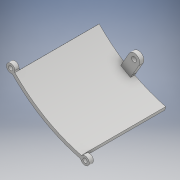
# Autodesk Inventor part: Wheel Guard1
Saved by Autodesk Inventor 2018 (Build 220112000, 112)
## iProperties
Created: 2017-10-13
Part Number: Wheel Guard1
Material: Generic
Document SubType Name: Modeling
Designer: BrisbaneMatt
Density: 1 g/cm^3
Appearance: Default
Author: BrisbaneMatt
Autodesk Inventor part; units mm, degrees
ref_plane "YZ Plane" through (0, 0, 0) normal (1, 0, 0) x (0, 1, 0)
ref_plane "XZ Plane" through (0, 0, 0) normal (0, 1, 0) x (-1, 0, 0)
ref_plane "XY Plane" through (0, 0, 0) normal (0, 0, 1) x (1, 0, 0)
sketch "Sketch1" plane through (0, 0, 0) normal (0, 1, 0) x (-1, 0, 0)
  circle A0 centre (0, 0) radius 100.151
  line L0 (0, 0) -> (50.0755, -86.7333)
  line L1 (0, 0) -> (100.151, 0) construction
  line L2 (0, 0) -> (50.0755, 86.7333)
  line L3 (0, 0) -> (100.151, 0) construction
  line L4 (0, 0) -> (-100.151, 0)
  line L5 (50.0755, -86.7333) -> (100.0755, -86.7333) construction
  line L6 (50.0755, -86.7333) -> (24.5339, -97.0995)
  line L7 (50.0755, -86.7333) -> (100.0755, -86.7333) construction
  line L8 (71.8237, -69.7967) -> (50.0755, -86.7333)
  circle A1 centre (0, 0) radius 102.651
  line L9 (0, 0) -> (71.8237, -69.7967)
  line L10 (71.8237, -69.7967) -> (73.6166, -71.539)
  line L11 (0, 0) -> (24.5339, -97.0995)
  line L12 (24.5339, -97.0995) -> (25.1463, -99.5233)
  dimension "d0" = 200.302
  dimension "d1" = 60
  dimension "d2" = 60
  dimension "d8" = 205.302
  constraints: 26 end point, 7 point on circle, 5 horizontal, 2 centre point, 2 coincident, 2 equal length, 2 point on line
  measures "d0" diameter of A0
  measures "d1" angle of L0 L1
  measures "d2" angle of L3 L2
  measures "d8" diameter of A1
extrude "Extrusion1" add sketch "Sketch1" along normal blind 40 contours L10 A1 L12 A0 picked at (67.2642, -76.2102)
sketch "Sketch2" plane through (0, 0, 0) normal (0, -1, 0) x (1, 0, 0)
  line L0 (-24.5339, -97.0995) -> (-25.1463, -99.5233) projected
  line L1 (-24.8401, -98.3114) -> (-21.9315, -99.0463)
  circle A0 centre (-21.9315, -99.0463) radius 1.5
  line L2 (-73.6166, -71.539) -> (-71.8237, -69.7967) projected
  line L3 (-72.7201, -70.6679) -> (-74.8716, -72.7586)
  line L4 (-74.8716, -72.7586) -> (-72.7201, -70.6679)
  line L5 (-72.7201, -70.6679) -> (-74.8109, -68.5164)
  circle A1 centre (-74.8109, -68.5164) radius 1.5
  circle A2 centre (-74.8109, -68.5164) radius 3
  arc A3 (-73.6166, -71.539) -> (-25.1463, -99.5233) centre (0, 0) ccw projected
  line L6 (-73.6166, -71.539) -> (-74.8109, -71.5164)
  arc A4 (-71.8237, -69.7967) -> (-24.5339, -97.0995) centre (0, 0) ccw projected
  line L7 (-71.8109, -68.5164) -> (-71.8237, -69.7967)
  circle A5 centre (-21.9315, -99.0463) radius 3
  line L8 (-21.9315, -99.0463) -> (-24.5296, -100.5463)
  line L9 (-21.9315, -99.0463) -> (-18.9315, -99.0463) construction
  line L10 (-24.5296, -100.5463) -> (-25.1463, -99.5233)
  arc A6 (-22.1585, -98.9889) -> (-21.9315, -99.0463) centre (-21.9315, -98.5684) ccw
  line L11 (-21.9315, -99.0463) -> (-22.9003, -97.4384)
  line L12 (-21.9315, -99.0463) -> (-20.0543, -99.0463) construction
  line L13 (-22.9003, -97.4384) -> (-23.4798, -96.4767)
  line L14 (-23.4798, -96.4767) -> (-24.5339, -97.0995)
  point P0 (0, 0)
  dimension "d12" = 3
  dimension "d13" = 3
  dimension "d14" = 3
  dimension "d15" = 210
  dimension "d16" = 121.07
  constraints: 26 end point, 8 point on circle, 5 centre point, 4 coincident, 2 collinear, 2 equal length, 2 horizontal, 2 midpoint, 2 point on line, 1 perpendicular, 1 tangent
  measures "d12" distance of L1.start L1.end
  measures "d13" distance of L3.start L3.end
  measures "d14" distance of L3.start L5.end
  measures "d16" angle of L12 L11
extrude "Extrusion2" add sketch "Sketch2" against normal blind 3 contours L14 A5 L0 | L7 L2 A2 | A5 L10 L0 | A5 L13 L11 A0 L1 | L1 A0 L8 A5 | A5 L8 A0 L11 L13 | A0 L11 L1 | L1 A6 L8 A0 | L2 L6 A2 | A2 | L1 A6 | A0 L8 L11
sketch "Sketch3" plane through (0, 3, 0) normal (0, 1, 0) x (1, 0, 0)
  arc A0 (-23.4798, 96.4767) -> (-24.5296, 100.5463) centre (-21.9315, 99.0463) ccw projected
  circle A1 centre (-21.9315, 99.0463) radius 1.5
  point P0 (0, 0)
  dimension "d19" = 3
  constraints: 1 centre point, 1 coincident
  measures "d19" diameter of A1
extrude "Extrusion3" cut sketch "Sketch3" against normal blind 3
sketch "Sketch4" plane through (-25.1463, 3, -99.5233) normal (0.9695, 0, -0.245) x (-0.245, 0, -0.9695)
  point P0 (-102.651, -3)
sketch "Sketch5" plane through (0, 40, 0) normal (0, 1, 0) x (1, 0, 0)
  circle A0 centre (-74.8109, 68.5164) radius 1.5 projected
  circle A1 centre (-21.9315, 99.0463) radius 1.5 projected
  line L0 (-74.8109, 68.5164) -> (-21.9315, 99.0463)
  circle A2 centre (-48.3712, 83.7814) radius 1.75
  circle A3 centre (-48.3712, 83.7814) radius 4
  line L1 (-44.9071, 85.7814) -> (-46.5714, 88.6641)
  arc A4 (-24.5339, 97.0995) -> (-71.8237, 69.7967) centre (0, 0) ccw projected
  line L2 (-51.8353, 81.7814) -> (-53.4996, 84.6641)
  line L3 (-46.5714, 88.6641) -> (-50.0755, 88.3957)
  line L4 (-50.0755, 88.3957) -> (-52.8557, 86.4967)
  line L5 (-52.8557, 86.4967) -> (-53.4996, 84.6641)
  point P0 (0, 0)
  dimension "d22" = 3.5
  dimension "d23" = 8
  constraints: 12 end point, 3 point on circle, 2 centre point, 2 point on line, 1 coincident, 1 midpoint, 1 parallel, 1 tangent
  measures "d22" diameter of A2
  measures "d23" diameter of A3
extrude "Extrusion4" add sketch "Sketch5" against normal blind 3 contours A3 A4 L0 A2 | L0 A2 A3 | L2 A4 A3 | L5 L4 L3 A4 A3 | A2 L0 | L0 A2 | A3 A4 | A3 A4 L1
sketch "Sketch6" plane through (0, 40, 0) normal (0, 1, 0) x (1, 0, 0)
  arc A0 (-51.8353, 81.7814) -> (-44.9071, 85.7814) centre (-48.3712, 83.7814) ccw projected
  circle A1 centre (-48.3712, 83.7814) radius 1.75
  point P0 (0, 0)
  dimension "d26" = 3.5
  constraints: 1 centre point, 1 coincident
  measures "d26" diameter of A1
extrude "Extrusion5" cut sketch "Sketch6" against normal blind 3
sketch "Sketch7" plane through (0, 40, 0) normal (0, 1, 0) x (1, 0, 0)
  point P0 (0, 0)
sketch "Sketch8" plane through (0, 40, 0) normal (0, 1, 0) x (1, 0, 0)
  line L0 (0, 0) -> (-59.2945, 80.7117)
  arc A0 (-53.4996, 84.6641) -> (-71.8237, 69.7967) centre (0, 0) ccw projected
  constraints: 2 end point, 1 point on circle
sketch "Sketch10" plane through (0, 40, 0) normal (0, 1, 0) x (1, 0, 0)
  circle A0 centre (-21.9315, 99.0463) radius 1.5 projected
  circle A1 centre (-74.8109, 68.5164) radius 1.5 projected
  line L0 (-21.9315, 99.0463) -> (-74.8109, 68.5164)
  line L1 (-48.3712, 83.7814) -> (0, 0)
  line L2 (-48.3712, 83.7814) -> (-44.0002, 76.2106)
  circle A2 centre (-44.0002, 76.2106) radius 1.75
  circle A3 centre (-44.0002, 76.2106) radius 4.01
  line L3 (-47.6057, 74.4556) -> (-52.7918, 83.4382)
  line L4 (-51.8353, 81.7814) -> (-53.4996, 84.6641) projected
  line L5 (-40.6779, 78.4561) -> (-45.4294, 86.686)
  line L6 (-45.4294, 86.686) -> (-49.4653, 86.686)
  line L7 (-49.4653, 86.686) -> (-52.7918, 83.4382)
  dimension "d30" = 96.7424
  dimension "d31" = 8.742
  dimension "d32" = 3.5
  constraints: 14 end point, 2 centre point, 2 coincident, 2 point on circle, 2 point on line, 1 horizontal, 1 midpoint, 1 parallel
  measures "d30" distance of L1.start L1.end
  measures "d31" distance of L1.start L2.end
  measures "d32" diameter of A2
extrude "Extrusion6" add sketch "Sketch10" along normal blind 20 and the other way blind 3 contours L5 A3 L1 L0 | L0 L3 L7 L6 L5 | L1 A3 L3 L0 | A3 L1 A2 | L1 A2 A3
sketch "Sketch11" plane through (0, 40, 0) normal (0, 1, 0) x (1, 0, 0)
  arc A0 (-24.5339, 97.0995) -> (-46.5714, 88.6641) centre (0, 0) ccw projected
  arc A1 (-24.5339, 97.0995) -> (-46.5714, 88.6641) centre (0, 0) ccw
  line L0 (-53.4996, 84.6641) -> (-52.7918, 83.4382) projected
  line L1 (-73.6166, 71.539) -> (-71.8237, 69.7967) projected
  arc A2 (-53.4996, 84.6641) -> (-71.8237, 69.7967) centre (0, 0) ccw
  arc A3 (-25.1463, 99.5233) -> (-73.6166, 71.539) centre (0, 0) ccw projected
  arc A4 (-25.1463, 99.5233) -> (-73.6166, 71.539) centre (0, 0) ccw
  line L2 (-25.1463, 99.5233) -> (-24.5339, 97.0995)
  line L3 (-73.6166, 71.539) -> (-71.8237, 69.7967)
  line L4 (-53.4996, 84.6641) -> (-52.7918, 83.4382)
  line L5 (-52.7918, 83.4382) -> (-49.4653, 86.686) projected
  line L6 (-52.7918, 83.4382) -> (-49.4653, 86.686)
  line L7 (-49.4653, 86.686) -> (-45.4294, 86.686) projected
  line L8 (-49.4653, 86.686) -> (-45.4294, 86.686)
  line L9 (-45.4294, 86.686) -> (-46.5714, 88.6641)
  point P0 (0, 0)
  dimension "d37" = 100.151
  constraints: 12 end point, 6 point on circle, 4 collinear, 3 centre point, 1 concentric
  measures "d37" radius of A2
extrude "Extrusion7" add sketch "Sketch11" along normal blind 20
sketch "Sketch12" plane through (0, 37, 0) normal (0, -1, 0) x (1, 0, 0)
  line L0 (-47.6057, -74.4556) -> (-53.4996, -84.6641) projected
  line L1 (-45.4294, -86.686) -> (-46.5714, -88.6641) projected
  arc A0 (-53.4996, -84.6641) -> (-46.5714, -88.6641) centre (0, 0) ccw
  line L2 (-53.4996, -84.6641) -> (-54.9814, -68.7673)
  line L3 (-54.9814, -68.7673) -> (-38.2505, -67.5322)
  line L4 (-38.2505, -67.5322) -> (-32.7507, -81.5808)
  line L5 (-32.7507, -81.5808) -> (-46.5714, -88.6641)
  point P0 (0, 0)
  constraints: 8 end point, 2 point on circle, 1 centre point
extrude "Extrusion8" cut sketch "Sketch12" against normal blind 20
body "Solid1"
